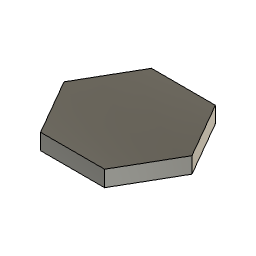
Hexagon (Autodesk Fusion 360 design; units mm, degrees)
Autodesk Fusion 360 part; units mm, degrees
sketch "Hexagon" plane through (0, 0, 0) normal (0, 0, 1) x (1, 0, 0)
  line L0 (6.35, 0) -> (0, -10.9985)
  line L1 (19.05, 0) -> (6.35, 0)
  line L2 (19.05, -21.9971) -> (25.4, -10.9985)
  line L3 (25.4, -10.9985) -> (19.05, 0)
  line L4 (0, -10.9985) -> (6.35, -21.9971)
  line L5 (6.35, -21.9971) -> (19.05, -21.9971)
extrude "Extrude1" add sketch "Hexagon" along normal blind 3.175
